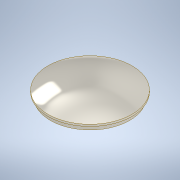
# Autodesk Inventor part: Tapadera
Saved by Autodesk Inventor 2020 (Build 240168000, 168)
## iProperties
Created: 2020-10-29
Part Number: Tapadera
Material: ABS Plastic
Document SubType Name: Modeling
Designer: aaron
Density: 1.06 g/cm^3
Appearance: Titanium - Polished
Author: aaron
Autodesk Inventor part; units mm, degrees
ref_plane "YZ Plane" through (0, 0, 0) normal (1, 0, 0) x (0, 1, 0)
ref_plane "XZ Plane" through (0, 0, 0) normal (0, 1, 0) x (-1, 0, 0)
ref_plane "XY Plane" through (0, 0, 0) normal (0, 0, 1) x (1, 0, 0)
sketch "Sketch1" plane through (0, 0, 0) normal (0, 1, 0) x (-1, 0, 0)
  circle A0 centre (0, 0) radius 45
  arc A1 (3.5, -41.3521) -> (-3.5, -41.3521) centre (0, 0) ccw
  circle A2 centre (0, 0) radius 42.5
  circle A3 centre (0, 0) radius 41.5
  point P0 (3.5, -41.3521)
  point P1 (-3.5, -41.3521)
  point P2 (3.5, -41.3521)
  point P3 (-3.5, -41.3521)
  dimension "d0" = 90
  dimension "d1" = 85
  dimension "d9" = 41.5
  constraints: 4 centre point, 3 coincident, 2 concentric, 2 point on circle
  measures "d0" diameter of A0
  measures "d1" diameter of A2
  measures "d9" radius of A1
extrude "Extrusion1" add sketch "Sketch1" along normal blind 2 contours A0
extrude "Extrusion2" add sketch "Sketch1" against normal blind 5 contours A2
sketch "Sketch2" plane through (0, 0, 0) normal (1, 0, 0) x (0, 1, 0)
  line L0 (0, 0) -> (9, 0)
  line L1 (2, -45) -> (2, 45) projected
  arc A0 (9, 0) -> (2, 45) centre (-120.9693, 2.827) ccw
  line L2 (9, 0) -> (7.5, 0)
  line L3 (2, 42.5) -> (0, 42.5) projected
  arc A1 (7.5, 0) -> (2, 42.5) centre (-116.3746, 5.5751) ccw
  line L4 (0, -63.0618) -> (0, 63.3707) projected
  line L5 (-147.3603, 0) -> (37.3769, 0) projected
  dimension "d14" = 9
  dimension "d15" = 130
  dimension "d16" = 1.5
  dimension "d17" = 124
  constraints: 4 end point, 4 point on circle, 3 point on line, 2 centre point, 1 horizontal
  measures "d14" distance of L0.start L0.end
  measures "d15" radius of A0
  measures "d16" distance of L0.end L2.end
  measures "d17" radius of A1
revolve "Revolution1" add sketch "Sketch2" angle 360 about axis through (0, -10, 0) along (0, 1, 0) contours A1 L1 A0 L0
body "Solid1"
